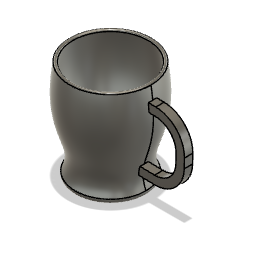
MUG (Autodesk Fusion 360 design; units mm, degrees)
Autodesk Fusion 360 part; units mm, degrees
sketch "Sketch1" plane through (0, 0, 0) normal (0, 0, 1) x (1, 0, 0)
  arc A0 (23.2572, 2.2665) -> (-23.2509, 2.197) centre (0.1336, -85.0801) ccw
  spline S0 degree 5 poles (23.4071, 2.4428) (23.0288, 3.197) (22.3522, 4.7448) (21.5772, 7.1846) (21.0318, 10.6776) (21.179, 15.4804) (22.1179, 20.7866) (23.679, 26.692) (25.5253, 33.319) (27.238, 40.8186) (28.3667, 49.3618) (28.4662, 57.1705) (27.9427, 63.6408) (27.3086, 68.2366) (26.9203, 70.605) knots 0 0 0 0 0 0 0.1 0.2 0.3 0.4 0.5 0.6 0.7 0.8 0.9 1 1 1 1 1 1
  line L0 (28.8401, 58.8956) -> (25.0005, 82.3145)
  spline S1 degree 3 poles (25.3594, 3.3138) (23.9392, 6.497) (23.2498, 9.6258) (23.2656, 12.8492) (23.2792, 15.6454) (23.8483, 18.5297) (24.8358, 21.8541) (25.9564, 25.6266) (27.6167, 29.967) (28.9082, 35.5314) (30.017, 40.3084) (30.8128, 45.9996) (30.7367, 53.0081) (30.68, 58.2256) (30.1403, 64.1786) (29.0299, 70.9509) knots 0.005493 0.005493 0.005493 0.005493 0.235384 0.235384 0.235384 0.434802 0.434802 0.434802 0.661099 0.661099 0.661099 0.855374 0.855374 0.855374 1 1 1 1
  arc A1 (22.7101, 0.2) -> (25.3594, 3.3138) centre (23.29, 2.3905) ccw
  arc A2 (22.7101, 0.2) -> (-22.6977, 0.1321) centre (0.1336, -85.0801) ccw
  arc A3 (23.2572, 2.2665) -> (23.4071, 2.4428) centre (23.29, 2.3905) ccw
  line L1 (-0.0014, 5.2754) -> (0.0018, 3.1376)
  arc A4 (29.0299, 70.9509) -> (26.9203, 70.605) centre (27.9751, 70.778) ccw
  point P0 (21.9105, 19.1701)
  constraint midpoint S0.end L0
  constraint concentric A0 A2
  constraint tangent A1 A2
  constraint tangent A0 A3
  constraint midpoint A0 L1.start
  constraint midpoint A2 L1.end
revolve "Revolve1" add sketch "Sketch1" angle 360 about axis through (-0.0014, 5.2754, 0) along (0.001494, -0.999999, 0)
sketch "Sketch2" plane through (0, 0, 0) normal (0, 0, 1) x (1, 0, 0)
  line L0 (-0.3234, 30.8314) -> (-0.0395, 44.6805)
  line L1 (18.3257, 62.3077) -> (35.4121, 61.9574)
  line L2 (55.9772, 40.5313) -> (55.8383, 33.7577)
  line L3 (34.4123, 13.1926) -> (12.7081, 13.6376)
  arc A0 (55.9772, 40.5313) -> (35.4121, 61.9574) centre (34.9816, 40.9618) ccw
  arc A1 (34.4123, 13.1926) -> (55.8383, 33.7577) centre (34.8427, 34.1882) ccw
  arc A2 (18.3257, 62.3077) -> (-0.0395, 44.6805) centre (17.9567, 44.3115) ccw
  arc A3 (-0.3234, 30.8314) -> (12.7081, 13.6376) centre (14.499, 28.5304) ccw
  line L4 (18.2027, 56.309) -> (35.2891, 55.9586)
  arc A4 (49.9785, 40.6543) -> (35.2891, 55.9586) centre (34.9816, 40.9618) ccw
  line L5 (49.9785, 40.6543) -> (49.8396, 33.8807)
  arc A5 (34.5352, 19.1914) -> (49.8396, 33.8807) centre (34.8427, 34.1882) ccw
  line L6 (34.5352, 19.1914) -> (12.6113, 19.6409)
  arc A6 (5.6752, 30.7044) -> (12.6113, 19.6409) centre (14.499, 28.5304) ccw
  line L7 (5.6752, 30.7044) -> (5.9593, 44.5575)
  arc A7 (18.2027, 56.309) -> (5.9593, 44.5575) centre (17.9567, 44.3115) ccw
  line L8 (26.8689, 62.1325) -> (26.7459, 56.1338)
  line L9 (18.0038, 19.5303) -> (17.8808, 13.5316)
  dimension "d8" = 21
  dimension "d9" = 18
  dimension "d10" = 15
  constraint perpendicular L0 L1
  constraint parallel L0 L2
  constraint parallel L1 L3
  constraint tangent L1 A0
  constraint tangent L2 A0
  constraint tangent L2 A1
  constraint tangent L3 A1
  constraint equal A0 A1
  constraint tangent L1 A2
  constraint tangent L0 A2
  constraint parallel L1 L4
  constraint concentric A0 A4
  constraint parallel L2 L5
  constraint concentric A1 A5
  constraint parallel L3 L6
  constraint concentric A3 A6
  constraint parallel L0 L7
  constraint concentric A2 A7
  constraint tangent L4 A7
  constraint tangent L4 A4
  constraint tangent A5 L6
  constraint midpoint L1 L8.start
  constraint midpoint L4 L8.end
  constraint coincident L6 L9.start
  constraint coincident L3 L9.end
  constraint perpendicular L3 L9
  measures "d8" radius of A0
  measures "d9" radius of A2
  measures "d10" radius of A3
extrude "Extrude1" add sketch "Sketch2" along normal mid plane 6 contours L1 L2 L3 A0 A1 L4 A4 L5 A5 L6 L8 L9
